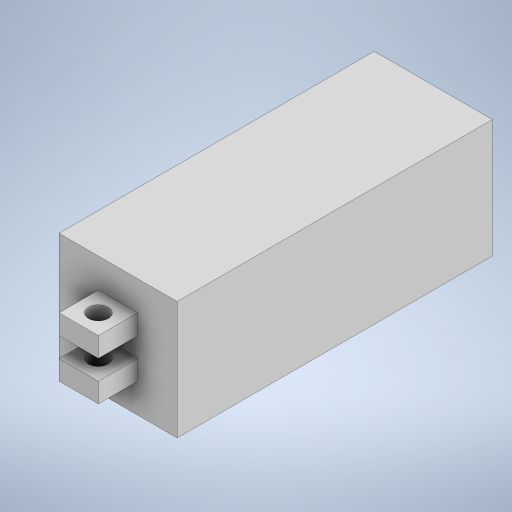
# Autodesk Inventor part: tail
Saved by Autodesk Inventor 2024 (Build 280153000, 153)
## iProperties
Created: 2023-10-17
Part Number: tail
Material: Generic
Document SubType Name: Modeling
Designer: Piter
Density: 1 g/cm^3
Appearance: Default
Author: Piter
Autodesk Inventor part; units mm, degrees
ref_plane "YZ Plane" through (0, 0, 0) normal (1, 0, 0) x (0, 1, 0)
ref_plane "XZ Plane" through (0, 0, 0) normal (0, 1, 0) x (-1, 0, 0)
ref_plane "XY Plane" through (0, 0, 0) normal (0, 0, 1) x (1, 0, 0)
sketch "Sketch1" plane through (0, 0, 0) normal (0, 1, 0) x (-1, 0, 0)
  line L0 (0, 0) -> (30, 0)
  line L1 (30, 0) -> (30, -80)
  line L2 (30, -80) -> (0, -80)
  line L3 (0, -80) -> (0, 0)
  dimension "d0" = 30
  dimension "d1" = 80
  constraints: 8 end point, 2 parallel, 1 horizontal, 1 perpendicular
  measures "d0" distance of L1.end L2.end
  measures "d1" distance of L0.end L1.end
extrude "Extrusion1" add sketch "Sketch1" along normal blind 30
sketch "Sketch2" plane through (-30, 0, 0) normal (0, 0, 1) x (1, 0, 0)
  line L0 (30, 0) -> (0, 0) projected
  line L1 (15, 0) -> (15, 7.5)
  line L2 (15, 7.5) -> (20, 7.5)
  line L3 (20, 7.5) -> (20, 12.5)
  line L4 (20, 12.5) -> (15, 12.5)
  line L5 (15, 12.5) -> (15, 7.5)
  line L6 (15, 12.5) -> (10, 12.5)
  line L7 (10, 12.5) -> (10, 7.5)
  line L8 (10, 7.5) -> (15, 7.5)
  line L9 (15, 7.5) -> (15, 12.5)
  line L10 (10, 12.5) -> (20, 12.5)
  line L11 (20, 12.5) -> (20, 17.5)
  line L12 (20, 17.5) -> (10, 17.5)
  line L13 (10, 17.5) -> (10, 12.5)
  line L14 (20, 17.5) -> (10, 17.5)
  line L15 (10, 17.5) -> (10, 22.5)
  line L16 (10, 22.5) -> (20, 22.5)
  line L17 (20, 22.5) -> (20, 17.5)
  dimension "d4" = 7.5
  dimension "d5" = 5
  dimension "d6" = 5
  dimension "d7" = 5
  dimension "d8" = 5
  dimension "d9" = 5
  dimension "d10" = 5
  constraints: 34 end point, 8 parallel, 4 horizontal, 4 perpendicular, 2 point on line, 1 midpoint, 1 vertical
  measures "d4" distance of L1.start L1.end
  measures "d5" distance of L4.end L3.end
  measures "d6" distance of L3.end L2.end
  measures "d7" distance of L8.end L7.end
  measures "d8" distance of L7.end L6.end
  measures "d9" distance of L11.end L10.end
  measures "d10" distance of L14.end L15.end
extrude "Extrusion2" add sketch "Sketch2" along normal blind 10 contours L5 L4 L3 L2 | L8 L7 L6 L5 | L12 L15 L16 L17
sketch "Sketch3" plane through (-20, 22.5, 0) normal (0, 1, 0) x (1, 0, 0)
  line L0 (0, 0) -> (0, -10) projected
  line L1 (0, -5) -> (10, -5)
  line L2 (10, 0) -> (10, -10) projected
  circle A0 centre (5, -5) radius 2.5
  point P0 (20, 0)
  dimension "d13" = 5
  constraints: 3 midpoint, 2 end point, 1 centre point
  measures "d13" diameter of A0
extrude "Extrusion3" cut sketch "Sketch3" against normal through all
sketch "Sketch4" plane through (0, 0, 0) normal (0, -1, 0) x (1, 0, 0)
  line L0 (-10, 0) -> (-20, 0) projected
  line L1 (-15, 0) -> (-15, -15)
  circle A0 centre (-15, -15) radius 2.5
  point P0 (0, 0)
  dimension "d16" = 15
  dimension "d17" = 5
  constraints: 2 end point, 1 centre point, 1 coincident, 1 midpoint, 1 vertical
  measures "d16" distance of L1.start L1.end
  measures "d17" diameter of A0
extrude "Extrusion4" cut sketch "Sketch4" against normal blind 5
body "Solid1"
